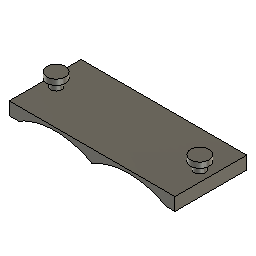
ADXL345 (Autodesk Fusion 360 archive; units mm, degrees)
design "Finger"
Autodesk Fusion 360 part; units mm, degrees
sketch "Sketch2" plane through (0, 0, 0) normal (0, 1, 0) x (1, 0, 0)
  line L0 (20, -1.5) -> (-20, -1.5)
  line L1 (-20, -1.5) -> (-20, 1.5)
  line L2 (-20, 1.5) -> (20, 1.5)
  line L3 (20, 1.5) -> (20, -1.5)
  line L4 (20, -1.5) -> (-20, 1.5) construction
  line L5 (-20, -1.5) -> (20, 1.5) construction
  line L6 (0, -1.5) -> (0, 1.5) construction
  arc A0 (-20, 1.5) -> (0, 1.5) centre (-10, 18.8205) ccw
  arc A1 (0, 1.5) -> (20, 1.5) centre (10, 18.8205) ccw
  line L7 (-20, 1.5) -> (-22.5, 1.5)
  line L8 (-22.5, 1.5) -> (-22.5, -1.5)
  line L9 (-22.5, -1.5) -> (-20, -1.5)
  line L10 (-20, -1.5) -> (-20, 1.5)
  line L11 (20, 1.5) -> (22.5, 1.5)
  line L12 (22.5, 1.5) -> (22.5, -1.5)
  line L13 (22.5, -1.5) -> (20, -1.5)
  line L14 (20, -1.5) -> (20, 1.5)
  dimension "d3" = 3
  dimension "d4" = 40
  dimension "d5" = 20
  dimension "d6" = 20
  dimension "d11" = 2.5
  dimension "d12" = 2.5
  constraint horizontal L0
  constraint perpendicular L0 L1
  constraint parallel L0 L2
  constraint parallel L1 L3
  constraint coincident L4 origin
  constraint coincident L5 origin
  constraint midpoint L0 L6.start
  constraint midpoint L2 L6.end
  constraint horizontal L7
  constraint vertical L8
  constraint horizontal L9
  constraint vertical L10
  constraint horizontal L11
  constraint vertical L12
  constraint horizontal L13
  constraint vertical L14
  constraint collinear L9 L13
  constraint collinear L0 L13
  measures "d3" distance of L0.end L1.end
  measures "d4" distance of L1.end L2.end
  measures "d5" radius of A0
  measures "d6" radius of A1
  measures "d11" distance of L2.end L11.end
  measures "d12" distance of L1.end L7.end
extrude "Extrude1" add sketch "Sketch2" along normal blind 19.5 contours L0 L1 L3 A0 A1 L10 L14 | L3 L11 L12 L13 L14 | L1 L7 L8 L9 L10
extrude "Extrude2" add 3 faces at (6.6667, 6.5, 1.5) (21.6667, 6.5, 1.5) (-21.6667, 6.5, 1.5) along direction (0, 0, 1) blind 0.5
sketch "Sketch3" plane through (0, 0, 2) normal (0, 0, 1) x (-1, 0, 0)
  line L0 (22.5, 0) -> (-22.5, 0)
  line L1 (-22.5, 0) -> (-22.5, -19.5)
  line L2 (-22.5, -19.5) -> (22.5, -19.5)
  line L3 (22.5, -19.5) -> (22.5, 0)
  line L4 (22.5, -9.75) -> (-22.5, -9.75) construction
  line L5 (0, -19.5) -> (0, 0) construction
  circle A0 centre (19.5, -9.75) radius 1.5
  dimension "d13" = 3
  dimension "d14" = 3
  constraint midpoint L3 L4.start
  constraint midpoint L1 L4.end
  constraint midpoint L2 L5.start
  constraint coincident L5.end origin
  constraint coincident L4 A0.centre
  measures "d13" diameter of A0
  measures "d14" distance of L3 A0.centre
extrude "Extrude3" add sketch "Sketch3" along normal blind 2 contours A0
sketch "Sketch4" plane through (0, 0, 4) normal (0, 0, 1) x (-1, 0, 0)
  circle A0 centre (19.5, -9.75) radius 1.5
  circle A1 centre (19.5, -9.75) radius 2.5
  dimension "d17" = 5
  constraint concentric A0 A1
  measures "d17" diameter of A1
extrude "Extrude4" add sketch "Sketch4" along normal blind 1.5 contours A0 | A1
ref_plane "WorkPlane1" through (0, 9.75, 0.25) normal (-1, 0, 0) x (0, 0, 1)
mirror "Mirror1" about plane through (0, 9.75, 0.25) normal (-1, 0, 0) of "Extrude3", "Extrude4"
equation "d7 = 16.5 mm + 3 mm"
